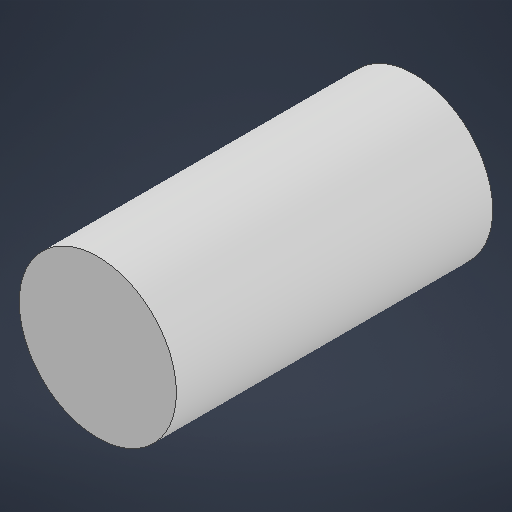
# Autodesk Inventor part: rim-v1
Saved by Autodesk Inventor 2026.2 (Build 302298010, 298A)
## iProperties
Created: 2026-05-11
Part Number: rim-v1
Material: Generic
Document SubType Name: Modeling
Designer: karol
Density: 1 g/cm^3
Appearance: Default
Author: karol
Autodesk Inventor part; units mm, degrees
ref_plane "YZ Plane" through (0, 0, 0) normal (1, 0, 0) x (0, 1, 0)
ref_plane "XZ Plane" through (0, 0, 0) normal (0, 1, 0) x (-1, 0, 0)
ref_plane "XY Plane" through (0, 0, 0) normal (0, 0, 1) x (1, 0, 0)
ref_plane "Work Plane1" through (0, 0, 0.5) normal (0, 0, 1) x (1, 0, 0)
sketch "Sketch1" plane through (0, 0, 0.5) normal (0, 0, 1) x (1, 0, 0)
  arc A0 (13, 1.882) -> (13, 4.118) centre (14, 3) ccw projected
  arc A1 (13, 1.882) -> (13, 4.118) centre (14, 3) ccw projected
  line L0 (13, 4.118) -> (13, 1.882) projected
  circle A2 centre (14, 3) radius 6
  circle A3 centre (14, 3) radius 4
  circle A4 centre (14, 3) radius 1.7
  line L1 (12.7, 1.9046) -> (12.7, 4.0954)
  point P0 (0, 0)
  dimension "d0" = 12
  dimension "d1" = 8
  dimension "d2" = 0.2
  dimension "d3" = 0.3
  constraints: 3 centre point, 3 coincident, 2 end point, 2 point on circle, 1 parallel, 1 vertical
  measures "d0" diameter of A2
  measures "d1" diameter of A3
  measures "d2" radial gap between concentric circles of A0 A4
  measures "d3" distance between parallel lines of L0 L1
extrude "Extrusion1" add sketch "Sketch1" along normal blind 21.5 contours A3 | L1 A4 picked at (12.5667, 3)
ref_plane "Work Plane2" through (14, 3, 18) normal (0, 0, 1) x (1, 0, 0)
sketch "Sketch2" plane through (14, 3, 18) normal (0, 0, 1) x (1, 0, 0)
  circle A0 centre (0, 0) radius 4 projected
  arc A1 (-1.3, -1.0954) -> (-1.3, 1.0954) centre (0, 0) ccw projected
  line L0 (-1.3, -1.0954) -> (-1.3, 1.0954) projected
  circle A2 centre (0, 0) radius 3
  point P0 (-14, -3)
  dimension "d7" = 6
  constraints: 1 centre point, 1 coincident
  measures "d7" diameter of A2
extrude "Extrusion2" cut sketch "Sketch2" against normal blind 2 contours A0
ref_plane "Work Plane3" through (9.7, 1.9046, 0.5) normal (1, 0, 0) x (0, 0, -1)
sketch "Sketch3" plane through (9.7, 1.9046, 0.5) normal (1, 0, 0) x (0, 0, -1)
  circle A0 centre (-2.5, 1) radius 1.5
  line L0 (-21.5, 0) -> (-21.5, 2.1909) projected
  point P0 (0.5, -1.9046)
  dimension "d11" = 3
  dimension "d12" = 1
  dimension "d15" = 19
  constraints: 1 centre point
  measures "d11" diameter of A0
  measures "d12" vertical distance of L0.start A0.centre
  measures "d15" distance from line of L0 A0.centre
extrude "Extrusion3" cut sketch "Sketch3" along normal blind 3.1
chamfer "Chamfer1" distance 0.25 angle 45 1 edges at (10.0014, 2.8924, 4.5)
ref_plane "Work Plane4" through (14, 3, 13) normal (0, 0, 1) x (1, 0, 0)
sketch "Sketch4" plane through (14, 3, 13) normal (0, 0, 1) x (1, 0, 0)
  circle A0 centre (0, 0) radius 4 projected
  circle A1 centre (0, 0) radius 4 projected
  circle A2 centre (0, 0) radius 3 projected
  point P0 (-14, -3)
extrude "Extrusion4" cut sketch "Sketch4" against normal blind 2
sketch "Sketch6" plane through (14, 3, 22) normal (0, 0, 1) x (1, 0, 0)
  circle A0 centre (0, 0) radius 3 projected
  circle A1 centre (0, 0) radius 6
  circle A2 centre (0, 0) radius 6.4
  point P0 (-14, -3)
  dimension "d22" = 12
  dimension "d23" = 12.8
  constraints: 2 centre point, 2 coincident
  measures "d22" diameter of A1
  measures "d23" diameter of A2
extrude "Extrusion5" add sketch "Sketch6" against normal blind 25 contours A2
extrude "Extrusion6" add sketch "Sketch6" along normal blind 0.8 contours A0 | A1 | A2
ref_plane "Płaszczyzna konstrukcyjna5" through (7.6, 1.9046, 0.5) normal (1, 0, 0) x (0, 0, -1)
sketch "Szkic7" plane through (7.6, 1.9046, 0.5) normal (1, 0, 0) x (0, 0, -1)
  spline S0 degree 5 poles (-1, 1) (-1, 1.1368) (-1.0156, 1.2734) (-1.0466, 1.4063) (-1.0917, 1.5328) (-1.205, 1.7681) (-1.2729, 1.8768) (-1.3508, 1.9761) (-1.4372, 2.0656) (-1.6936, 2.2827) (-1.8782, 2.3897) (-2.0794, 2.4628) (-2.2897, 2.5) (-2.7515, 2.5) (-3.0029, 2.4467) (-3.2389, 2.3425) (-3.4475, 2.1913) (-3.7919, 1.8049) (-3.9265, 1.5707) (-4.0157, 1.2926) (-4.0258, 0.9956) (-3.9322, 0.5012) (-3.8503, 0.294) (-3.7361, 0.1132) (-3.5976, -0.0424) (-3.2801, -0.2973) (-3.1013, -0.3969) (-2.9068, -0.4652) (-2.7034, -0.5) (-2.2715, -0.5) (-2.0431, -0.456) (-1.8272, -0.37) (-1.6331, -0.2455) (-1.3913, -0.0156) (-1.3217, 0.0629) (-1.2585, 0.148) (-1.2025, 0.2396) (-1.0957, 0.4562) (-1.0489, 0.5848) (-1.0164, 0.7201) (-1, 0.8595) (-1, 1) knots 0 0 0 0 0 0 0.066866 0.066866 0.066866 0.066866 0.133732 0.133732 0.133732 0.133732 0.249889 0.249889 0.249889 0.249889 0.388807 0.388807 0.388807 0.388807 0.527724 0.527724 0.527724 0.527724 0.638915 0.638915 0.638915 0.638915 0.750105 0.750105 0.750105 0.750105 0.875003 0.875003 0.875003 0.875003 0.931327 0.931327 0.931327 0.931327 1 1 1 1 1 1 projected
  point P0 (0.5, -1.9046)
  constraints: 2 other
extrude "Wyciągnięcie proste7" cut sketch "Szkic7" along normal blind 1
body "Solid1"
